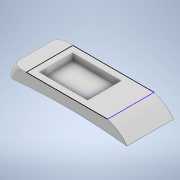
# Autodesk Inventor part: Case - Bottom
Saved by Autodesk Inventor 2020 (Build 240168000, 168)
## iProperties
Created: 2019-07-11
Part Number: Case - Bottom
Material: Generic
Document SubType Name: Modeling
Designer: tyrre
Density: 1 g/cm^3
Appearance: Default
Author: tyrre
Autodesk Inventor part; units mm, degrees
ref_plane "YZ Plane" through (0, 0, 0) normal (1, 0, 0) x (0, 1, 0)
ref_plane "XZ Plane" through (0, 0, 0) normal (0, 1, 0) x (-1, 0, 0)
ref_plane "XY Plane" through (0, 0, 0) normal (0, 0, 1) x (1, 0, 0)
sketch "Sketch1" plane through (0, 0, 0) normal (0, 0, 1) x (1, 0, 0)
  line L0 (-31.035, -5.2) -> (31.035, -5.2)
  line L1 (31.035, -5.2) -> (31.035, 5.2)
  line L2 (31.035, 5.2) -> (-31.035, 5.2)
  line L3 (-31.035, 5.2) -> (-31.035, -5.2)
  line L4 (-31.035, -5.2) -> (31.035, 5.2) construction
  line L5 (31.035, -5.2) -> (-31.035, 5.2) construction
  point P0 (0, 0)
  dimension "d0" = 62.07
  dimension "d1" = 10.4
  constraints: 12 end point, 2 midpoint, 2 parallel, 1 horizontal, 1 perpendicular
  measures "d0" distance of L2.end L1.end
  measures "d1" distance of L1.end L0.end
extrude "Extrusion1" add sketch "Sketch1" along normal mid plane 35.5
sketch "Sketch2" plane through (-31.035, 5.2, 17.75) normal (0, 1, 0) x (1, 0, 0)
  line L0 (0, 0) -> (0, 35.5) projected
  line L1 (0, 0) -> (0, 5)
  line L2 (0, 5) -> (5, 5)
  line L3 (5, 5) -> (5, 30.5)
  line L4 (5, 30.5) -> (42, 30.5)
  line L5 (42, 30.5) -> (42, 5)
  line L6 (42, 5) -> (5, 5)
  point P0 (31.035, 17.75)
  dimension "d4" = 5
  dimension "d5" = 5
  dimension "d6" = 25.5
  dimension "d7" = 37
  constraints: 12 end point, 2 parallel, 1 horizontal, 1 perpendicular, 1 point on line, 1 vertical
  measures "d4" distance of L0.start L1.end
  measures "d5" distance of L1.end L2.end
  measures "d6" distance of L2.end L3.end
  measures "d7" distance of L3.end L4.end
extrude "Extrusion2" cut sketch "Sketch2" against normal blind 5.2
sketch "Sketch3" plane through (0, 0, 17.75) normal (0, 0, 1) x (1, 0, 0)
  line L0 (31.035, -5.2) -> (-31.035, -5.2) projected
  point P0 (0, 0)
  point P1 (0, -2.6)
sketch "Sketch4" plane through (31.035, -5.2, 17.75) normal (1, 0, 0) x (0, 0, -1)
  line L0 (35.5, 0) -> (0, 0) projected
  line L1 (0, 10.4) -> (35.5, 10.4)
  line L2 (35.5, 10.4) -> (35.5, 0)
  line L3 (35.5, 0) -> (0, 0)
  line L4 (0, 0) -> (0, 10.4)
  line L5 (0, 10.4) -> (35.5, 0) construction
  line L6 (35.5, 10.4) -> (0, 0) construction
  point P0 (17.75, 5.2)
  constraints: 12 end point, 2 midpoint, 2 parallel, 1 horizontal, 1 perpendicular
extrude "Extrusion3" add sketch "Sketch4" along normal blind 15 separate body
sketch "Sketch5" plane through (31.035, -5.2, 17.75) normal (0, 0, 1) x (1, 0, 0)
  line L0 (0, 0) -> (0, 10.4) projected
  arc A0 (15, 0) -> (0, 10.4) centre (-7.2491, -16.0727) ccw
  line L1 (15, 0) -> (15, 10.4) projected
  line L2 (0, 10.4) -> (15, 10.4)
  line L3 (15, 10.4) -> (15, 0)
  point P0 (-31.035, 5.2)
  constraints: 4 end point, 2 point on circle, 1 centre point, 1 horizontal, 1 perpendicular
extrude "Extrusion4" cut sketch "Sketch5" against normal through all bodies 2
mirror "Mirror1" about plane through (0, 0, 0) normal (1, 0, 0) bodies 2
combine bodies "Combine1" operation type add bodies to combine 2 1
sketch "Sketch7" plane through (-46.035, -5.2, 17.75) normal (0, 0, 1) x (1, 0, 0)
  line L0 (92.07, 0) -> (0, 0) projected
  arc A0 (92.07, 0) -> (0, 0) centre (46.035, -395.5005) ccw
  point P0 (46.035, 5.2)
  point P1 (0, 0)
  constraints: 2 point on circle, 1 centre point
extrude "Extrusion5" cut sketch "Sketch7" against normal through all bodies 2
sketch "Sketch8" plane through (-31.035, 5.2, 17.75) normal (0, 1, 0) x (1, 0, 0)
  line L0 (0, 35.5) -> (0, 0) projected
  line L1 (0, 35.5) -> (0, 0)
  line L2 (0, 0) -> (62.07, 0)
  line L3 (62.07, 0) -> (62.07, 35.5)
  line L4 (62.07, 35.5) -> (0, 35.5)
  point P0 (31.035, 17.75)
  constraints: 8 end point, 2 parallel, 1 perpendicular, 1 vertical
sketch "Sketch9" plane through (-31.035, 5.2, 17.75) normal (0, 0, 1) x (1, 0, 0)
  arc A0 (77.07, -10.4) -> (-15, -10.4) centre (31.035, -405.9005) ccw projected
  line L0 (0, 0) -> (-15, 0)
  line L1 (-15, 0) -> (-15, -10.4)
  line L2 (-15, -10.4) -> (0, -10.4)
  line L3 (0, -10.4) -> (0, 0)
  point P0 (31.035, -5.2)
  point P1 (0, -8.9412)
  constraints: 8 end point, 2 parallel, 1 horizontal, 1 perpendicular, 1 point on circle
extrude "Extrusion6" add sketch "Sketch9" against normal blind 35.5 contours A0 L1 L0 L3 bodies 2
sketch "Sketch10" plane through (31.035, 5.2, 17.75) normal (0, 1, 0) x (1, 0, 0)
  line L0 (-57.07, 30.5) -> (-20.07, 30.5) projected
  line L1 (-20.07, 30.5) -> (-20.07, 5) projected
  line L2 (-20.07, 5) -> (-57.07, 5) projected
  line L3 (-57.07, 5) -> (-57.07, 30.5) projected
  line L4 (0, 0) -> (-77.07, 0) projected
  line L5 (0, 35.5) -> (0, 0) projected
  line L6 (-77.07, 35.5) -> (0, 35.5) projected
  line L7 (-77.07, 0) -> (-77.07, 35.5) projected
  line L8 (0, 0) -> (-77.07, 0) projected
  line L9 (-62.0537, 0) -> (-77.07, 0)
  line L10 (-77.07, 0) -> (-77.07, 35.5)
  line L11 (-77.07, 35.5) -> (-62.0537, 35.5)
  line L12 (-62.0537, 35.5) -> (-62.0537, 0)
  point P0 (-31.035, 17.75)
  constraints: 8 end point, 2 parallel, 1 collinear, 1 perpendicular, 1 point on line
extrude "Extrusion7" add sketch "Sketch10" along normal blind 7.5 contours L4 L7 L6 L12 bodies 2
sketch "Sketch11" plane through (0, -400.7005, 17.75) normal (0, 0, 1) x (1, 0, 0)
  line L0 (-31.0187, 405.9005) -> (-31.0187, 413.4005) projected
  arc A0 (-31.0187, 413.4005) -> (-46.035, 395.5005) centre (-24.2448, 392.4693) ccw
  line L1 (-46.035, 395.5005) -> (-46.035, 413.4005)
  line L2 (-46.035, 413.4005) -> (-31.0187, 413.4005) projected
  line L3 (-46.035, 413.4005) -> (-31.0187, 413.4005)
  point P0 (0, 400.7005)
  dimension "d21" = 22
  constraints: 4 end point, 2 point on circle, 1 centre point, 1 perpendicular, 1 vertical
  measures "d21" radius of A0
extrude "Extrusion8" cut sketch "Sketch11" against normal through all bodies 2
sketch "Sketch12" plane through (-31.0187, 5.2, 17.75) normal (0, 0, 1) x (1, 0, 0)
  line L0 (0, 0) -> (0, 7.5) projected
  line L1 (0, 0) -> (0, 7.5)
  line L2 (0, 7.5) -> (-11.3188, 7.5)
  line L3 (-11.3188, 7.5) -> (-11.3188, 0)
  line L4 (-11.3188, 0) -> (0, 0)
  point P0 (31.0187, -5.2)
  constraints: 8 end point, 3 equal length, 1 perpendicular
extrude "Extrusion9" cut sketch "Sketch12" against normal through all bodies 2
fillet "Fillet1" radius 5 2 edges at (-44.5298, 0.2846, 17.75) (-44.5298, 0.2846, -17.75)
body "Solid2"
